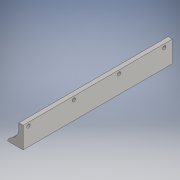
# Autodesk Inventor part: Intake inclined edge bottom
Saved by Autodesk Inventor 2016 (Build 200138000, 138)
## iProperties
Created: 2016-11-20
Part Number: Intake inclined edge bottom
Material: Generic
Document SubType Name: Modeling
Designer: paul_
Density: 1 g/cm^3
Appearance: Default
Author: paul_
Autodesk Inventor part; units mm, degrees
ref_plane "YZ Plane" through (0, 0, 0) normal (1, 0, 0) x (0, 1, 0)
ref_plane "XZ Plane" through (0, 0, 0) normal (0, 1, 0) x (-1, 0, 0)
ref_plane "XY Plane" through (0, 0, 0) normal (0, 0, 1) x (1, 0, 0)
sketch "Sketch1" plane through (0, 0, 0) normal (0, 0, 1) x (1, 0, 0)
  line L0 (-5.0917, 19.05) -> (-5.0917, 25.4)
  line L1 (0, 25.4) -> (-5.0917, 25.4)
  line L2 (-18.4964, 0) -> (0, 0)
  line L3 (0, 25.4) -> (0, 0)
  arc A0 (-12.7, 6.35) -> (-5.0917, 19.05) centre (-19.7746, 19.2173) ccw
  spline S0 degree 2 poles (-12.7, 6.35) (-18.092, 3.6812) (-18.4964, 0) knots 0 0 0 1 1 1
  point P0 (-17.2168, 2.9909)
  dimension "d1" = 6.35
  dimension "d7" = 25.4
  dimension "d8" = 18.4964
  constraints: 8 end point, 2 horizontal, 2 point on circle, 1 centre point, 1 vertical, 3 other
  measures "d1" distance of L0.start L0.end
  measures "d7" distance of L1.start L2.end
  measures "d8" distance of L2.start L2.end
extrude "Extrusion1" add sketch "Sketch1" along normal blind 177.8
hole "Hole1" at (0, 21.4671, 171.3774) direction (-1, 0, 0) diameter 4 end through all
pattern_linear "Rectangular Pattern1" count 4 spacing 53.848 along (0, 0, -1) of "Hole1"
body "Solid1"
